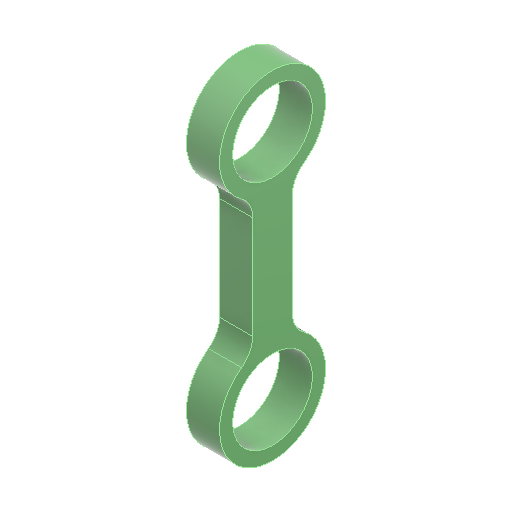
# Autodesk Inventor part: Link_GH
Saved by Autodesk Inventor 2026.2 (Build 302298000, 298)
## iProperties
Created: 2025-12-27
Part Number: Link_GH
Material: ABS 塑膠
Document SubType Name: Modeling
Designer: Hsiangyu
Density: 1.06 g/cm^3
Appearance: 平滑 - 深森林綠
Author: Hsiangyu
Autodesk Inventor part; units mm, degrees
ref_plane "YZ Plane" through (0, 0, 0) normal (1, 0, 0) x (0, 1, 0)
ref_plane "XZ Plane" through (0, 0, 0) normal (0, 1, 0) x (-1, 0, 0)
ref_plane "XY Plane" through (0, 0, 0) normal (0, 0, 1) x (1, 0, 0)
sketch "草圖1" plane through (0, 0, 0) normal (1, 0, 0) x (0, 1, 0)
  line L0 (0, 0) -> (-35, 0)
  circle A0 centre (0, 0) radius 6
  circle A1 centre (-35, 0) radius 6
  circle A2 centre (0, 0) radius 8
  circle A3 centre (-35, 0) radius 8
  line L1 (-7.4162, 3) -> (-27.5838, 3)
  line L2 (-27.5838, -3) -> (-7.4162, -3)
  dimension "d0" = 35
  dimension "d1" = 12
  dimension "d2" = 12
  dimension "d3" = 16
  dimension "d4" = 16
  dimension "d5" = 3
  dimension "d6" = 3
  constraints: 6 end point, 4 centre point, 4 coincident, 4 point on circle, 3 horizontal
  measures "d0" distance of L0.start L0.end
  measures "d1" diameter of A0
  measures "d2" diameter of A1
  measures "d3" diameter of A2
  measures "d4" diameter of A3
  measures "d5" distance between parallel lines of L1 L0
  measures "d6" distance between parallel lines of L0 L2
extrude "擠出1" add sketch "草圖1" along normal mid plane 5
fillet "圓角1" radius 4 4 edges at (0, -7.4162, 3) (0, -27.5838, 3) (0, -7.4162, -3) (0, -27.5838, -3)
equation "\"d2\" = d1"
equation "\"d4\" = d3"
equation "\"d6\" = d5"
